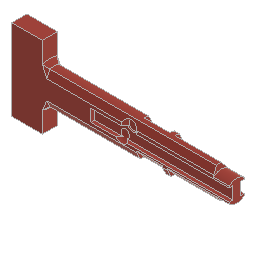
protec (Autodesk Fusion 360 design; units mm, degrees)
Autodesk Fusion 360 part; units mm, degrees
note: some values were not read from the file. Chosen so that the rebuilt part matches the saved one: which face or edge a step refers to; which pieces of a blend or face edit are solid.
sketch "profile" plane through (0, 0, 0) normal (1, 0, 0) x (0, 1, 0)
  line L0 (0, 0) -> (3.3, 0) construction
  line L1 (3.3, 0) -> (3.3, 3.3) construction
  line L2 (3.3, 3.3) -> (4.05, 3.3) construction
  line L3 (3.3, 3.3) -> (2.55, 3.3) construction
  line L4 (4.05, 3.3) -> (4.05, 4.5)
  line L5 (2.55, 3.3) -> (2.55, 2.1)
  line L6 (4.05, 3.3) -> (4.05, 2.1)
  line L7 (2.55, 3.3) -> (2.55, 4.5)
  line L8 (4.05, 4.5) -> (4.775, 4.5)
  line L9 (2.55, 2.1) -> (1.825, 2.1)
  line L10 (4.05, 2.1) -> (4.775, 2.1)
  line L11 (2.55, 4.5) -> (1.825, 4.5)
  line L12 (4.775, 4.5) -> (4.775, 5.165)
  line L13 (1.825, 2.1) -> (1.825, 1.435)
  line L14 (1.825, 4.5) -> (1.825, 5.165)
  line L15 (4.775, 2.1) -> (4.775, 1.435)
  line L16 (4.775, 5.165) -> (4.1589, 6.4863)
  line L17 (4.775, 5.165) -> (3.3, 5.165) construction
  line L18 (1.825, 1.435) -> (2.4411, 0.1137)
  line L19 (1.825, 5.165) -> (2.4411, 6.4863)
  line L20 (1.825, 5.165) -> (3.3, 5.165) construction
  line L21 (4.775, 1.435) -> (4.1589, 0.1137)
  arc A0 (4.1589, 6.4863) -> (2.4411, 6.4863) centre (3.3, 3.3) ccw
  arc A1 (2.4411, 0.1137) -> (4.1589, 0.1137) centre (3.3, 3.3) ccw
  dimension "d64" = 3.3
  dimension "d65" = 3.3
  dimension "d66" = 0.75
  dimension "d67" = 0.75
  dimension "d68" = 1.2
  dimension "d69" = 1.2
  dimension "d70" = 1.2
  dimension "d71" = 1.2
  dimension "d72" = 0.725
  dimension "d73" = 0.725
  dimension "d74" = 0.725
  dimension "d75" = 0.725
  dimension "d76" = 65
  dimension "d77" = 65
  dimension "d78" = 4.25
  dimension "d79" = 4.25
  dimension "d80" = 3.3
  constraint coincident L0.start origin
  constraint horizontal L0
  constraint perpendicular L0 L1
  constraint perpendicular L1 L2
  constraint perpendicular L1 L3
  constraint perpendicular L2 L4
  constraint perpendicular L3 L5
  constraint perpendicular L2 L6
  constraint perpendicular L3 L7
  constraint perpendicular L4 L8
  constraint perpendicular L5 L9
  constraint perpendicular L6 L10
  constraint perpendicular L7 L11
  constraint perpendicular L8 L12
  constraint perpendicular L9 L13
  constraint equal L12 L13
  constraint perpendicular L11 L14
  constraint perpendicular L10 L15
  constraint equal L14 L15
  constraint horizontal L17
  constraint vertical L1.end L17.end
  constraint equal L16 L18
  constraint parallel L16 L18
  constraint horizontal L20
  constraint parallel L19 L21
  constraint equal L19 L21
  constraint coincident L1.end L2.start
  constraint coincident L16.end A0.start
  measures "d64" distance of L0.start L0.end
  measures "d65" distance of L0.end L1.end
  measures "d66" distance of L1.end L2.end
  measures "d67" distance of L1.end L3.end
  measures "d68" distance of L2.end L4.end
  measures "d69" distance of L3.end L5.end
  measures "d70" distance of L2.end L6.end
  measures "d71" distance of L3.end L7.end
  measures "d72" distance of L4.end L8.end
  measures "d73" distance of L5.end L9.end
  measures "d74" distance of L6.end L10.end
  measures "d75" distance of L7.end L11.end
  measures "d76" angle of L16 L17
  measures "d77" angle of L19 L20
  measures "d78" distance of L16 L18
  measures "d79" distance of L19 L21
  measures "d80" radius of A0
extrude "Extrude1" add sketch "profile" against normal blind 42.57 makes body 1
ref_plane "WorkPlane1" through (-21.285, 3.3, 3.3) normal (0, -1, 0) x (0, 0, 1)
ref_plane "WorkPlane2" through (-42.57, 0, 0) normal (1, 0, 0) x (0, 1, 0)
sketch "bow" plane through (-42.57, 0, 0) normal (1, 0, 0) x (0, 1, 0)
  line L0 (2.55, 2.1) -> (2.55, 4.5)
  line L1 (2.55, 4.5) -> (1.825, 4.5)
  line L2 (1.825, 4.5) -> (1.825, 5.165) construction
  line L3 (1.825, 5.165) -> (2.4411, 6.4863) construction
  arc A0 (4.1589, 6.4863) -> (2.4411, 6.4863) centre (3.3, 3.3) ccw construction
  line L4 (4.1589, 6.4863) -> (4.775, 5.165) construction
  line L5 (4.775, 5.165) -> (4.775, 4.5) construction
  line L6 (4.775, 4.5) -> (4.05, 4.5)
  line L7 (4.05, 4.5) -> (4.05, 2.1)
  line L8 (4.05, 2.1) -> (4.775, 2.1)
  line L9 (4.775, 2.1) -> (4.775, 1.435) construction
  line L10 (4.775, 1.435) -> (4.1589, 0.1137) construction
  arc A1 (2.4411, 0.1137) -> (4.1589, 0.1137) centre (3.3, 3.3) ccw construction
  line L11 (2.4411, 0.1137) -> (1.825, 1.435) construction
  line L12 (1.825, 1.435) -> (1.825, 2.1) construction
  line L13 (1.825, 2.1) -> (2.55, 2.1)
  circle A2 centre (3.3, 3.3) radius 3.3 construction
  line L14 (1.825, 5.165) -> (1.825, 6.252)
  line L15 (1.825, 1.435) -> (1.825, 0.348)
  line L16 (4.775, 1.435) -> (4.775, 0.348)
  line L17 (4.775, 5.165) -> (4.775, 6.252)
  line L18 (1.825, 2.1) -> (1.825, 4.5)
  line L19 (4.775, 4.5) -> (4.775, 2.1)
  line L20 (1.825, 6.252) -> (1.825, 11.252)
  line L21 (4.775, 0.348) -> (4.775, -4.652)
  line L22 (1.825, 11.252) -> (4.775, 11.252)
  line L23 (4.775, 11.252) -> (4.775, 6.252)
  line L24 (4.775, -4.652) -> (1.825, -4.652)
  line L25 (1.825, -4.652) -> (1.825, 0.348)
  line L26 (1.825, 1.435) -> (1.825, 2.1)
  line L27 (4.775, 2.1) -> (4.775, 1.435)
  line L28 (4.775, 5.165) -> (4.775, 4.5)
  line L29 (1.825, 5.165) -> (1.825, 4.5)
  dimension "d84" = 5
  constraint concentric A0 A2
  constraint coincident L3.end A2
  constraint coincident L2.end L3.start
  constraint coincident A2 L14.end
  constraint parallel L2 L14
  constraint coincident L11.end L12.start
  constraint coincident A2 L15.end
  constraint parallel L12 L15
  constraint coincident L9.end L10.start
  constraint coincident A2 L16.end
  constraint parallel L9 L16
  constraint coincident L4.end L5.start
  constraint coincident A2 L17.end
  constraint parallel L5 L17
  constraint coincident L12.end L13.start
  constraint coincident L1.end L2.start
  constraint coincident L5.end L6.start
  constraint coincident L8.end L9.start
  constraint parallel L14 L20
  constraint parallel L16 L21
  constraint equal L20 L21
  constraint perpendicular L17 L22
  constraint perpendicular L22 L23
  constraint perpendicular L15 L24
  constraint perpendicular L24 L25
  measures "d84" distance of L14.end L20.end
sketch "dss holes + dc align" plane through (0, 3.3, 0) normal (0, -1, 0) x (-1, 0, 0)
  line L0 (0, -4.5) -> (0, -2.1) construction
  line L1 (0, -3.3) -> (19.57, -3.3) construction
  line L2 (19.57, -3.3) -> (21.07, -3.3) construction
  line L3 (19.57, -3.3) -> (19.57, -4.9) construction
  line L4 (19.57, -3.3) -> (19.57, -1.7) construction
  line L5 (21.07, -3.3) -> (21.07, -4.1) construction
  line L6 (21.07, -3.3) -> (21.07, -2.5) construction
  circle A0 centre (19.57, -4.9) radius 0.9
  circle A1 centre (16.57, -4.9) radius 0.9
  circle A2 centre (19.57, -1.7) radius 0.9
  circle A3 centre (16.57, -1.7) radius 0.9
  dimension "d85" = 19.57
  dimension "d86" = 1.5
  dimension "d87" = 1.6
  dimension "d88" = 0.8
  dimension "d89" = 1.8
  dimension "d90" = 3
  constraint midpoint L0 L1.start
  constraint perpendicular L0 L1
  constraint parallel L1 L2
  constraint perpendicular L2 L3
  constraint perpendicular L2 L4
  constraint equal L3 L4
  constraint perpendicular L2 L5
  constraint perpendicular L2 L6
  constraint equal L5 L6
  constraint coincident L3.end A0.centre
  constraint equal A0 A1
  constraint horizontal L3.end A1.centre
  constraint symmetric L1 A0 A2
  constraint symmetric L1 A1 A3
  measures "d85" distance of L1.start L1.end
  measures "d86" distance of L1.end L2.end
  measures "d87" distance of L1.end L3.end
  measures "d88" distance of L2.end L5.end
  measures "d89" diameter of A0
  measures "d90" distance of L3.end A1.centre
ref_plane "WorkPlane3" through (-21.07, 0, 0) normal (1, 0, 0) x (0, 1, 0)
sketch "dc bearings" plane through (-21.07, 0, 0) normal (1, 0, 0) x (0, 1, 0)
  line L0 (0, 0) -> (3.3, 0) construction
  line L1 (3.3, 0) -> (3.3, 3.3) construction
  line L2 (3.3, 3.3) -> (1.4542, 2.8398) construction
  line L3 (3.3, 3.3) -> (1.4542, 3.3) construction
  circle A0 centre (1.4542, 2.8398) radius 1.375
  line L4 (3.3, 3.3) -> (5.1458, 3.7602) construction
  circle A1 centre (5.1458, 3.7602) radius 1.375
  dimension "d92" = 3.3
  dimension "d93" = 3.3
  dimension "d94" = 14
  dimension "d95" = 1.9023
  dimension "d96" = 2.75
  constraint coincident L0.start origin
  constraint horizontal L0
  constraint perpendicular L0 L1
  constraint horizontal L3
  constraint coincident L2.end A0.centre
  constraint vertical L3.end L2.end
  constraint parallel L2 L4
  constraint equal L2 L4
  constraint coincident L4.end A1.centre
  constraint equal A0 A1
  measures "d92" distance of L0.start L0.end
  measures "d93" distance of L0.end L1.end
  measures "d94" angle of L2 L3
  measures "d95" distance of L1.end L2.end
  measures "d96" diameter of A0
extrude "Extrude2" add sketch "bow" along normal blind 6 bodies 1
extrude "Extrude3" add 2 faces at (-36.57, 2.0667, 3.7) (-36.57, 4.5333, 2.9) along direction (1, 0, 0) blind 9.5 on bodies 1 bodies 1
chamfer "Chamfer1" distance 0.85 angle 45 6 edges at (-36.57, 4.4669, 5.8256) (-36.57, 3.3, 6.6) (-36.57, 2.1331, 5.8256) (-36.57, 2.1331, 0.7744) (-36.57, 3.3, 0) (-36.57, 4.4669, 0.7744) on bodies 1
extrude "Extrude4" add sketch "dc bearings" along normal mid plane 2.75 separate body makes body 2 at (-20.1533, 6.5191, 3.6917) makes body 3 at (-20.1533, 2.8275, 2.7712)
fillet "Fillet1" radius 1.375 4 edges at (-19.695, 3.7708, 3.7602) (-22.445, 3.7708, 3.7602) (-19.695, 0.0792, 2.8398) (-22.445, 0.0792, 2.8398) on bodies 2 3
combine "Combine1" operation cut target body 1 tool bodies 2 3
extrude "Extrude5" cut sketch "dss holes + dc align" along normal blind 0.9 draft 35 from surface at 0.575 contours A0 bodies 1
extrude "Extrude6" cut sketch "dss holes + dc align" against normal blind 0.9 draft 35 from surface at -0.575 contours A2 bodies 1
extrude "Extrude17" [suppressed]
extrude "Extrude18" [suppressed]
sketch "profiled 0 cut" plane through (0, 0, 0) normal (1, 0, 0) x (0, 1, 0)
  line L0 (2.55, 4.5) -> (1.825, 4.5)
  line L1 (2.55, 3.3) -> (2.55, 4.5)
  line L2 (2.55, 3.3) -> (2.55, 2.1)
  line L3 (2.55, 2.1) -> (1.825, 2.1)
  line L4 (4.05, 3.3) -> (4.05, 2.1)
  line L5 (4.05, 2.1) -> (4.775, 2.1)
  line L6 (4.05, 3.3) -> (4.05, 4.5)
  line L7 (4.05, 4.5) -> (4.775, 4.5)
  line L8 (4.775, 4.5) -> (4.775, 4.8293)
  line L9 (1.825, 2.1) -> (1.825, 1.7707)
  line L10 (1.825, 4.5) -> (1.825, 4.8293)
  line L11 (4.775, 2.1) -> (4.775, 1.7707)
  line L12 (4.775, 4.8293) -> (4.7747, 4.83)
  line L13 (4.775, 4.8293) -> (3.3, 4.8293) construction
  line L14 (1.825, 1.7707) -> (1.8253, 1.77)
  line L15 (1.825, 4.8293) -> (1.8253, 4.83)
  line L16 (1.825, 4.8293) -> (3.3, 4.8293) construction
  line L17 (4.775, 1.7707) -> (4.7747, 1.77)
  arc A0 (4.7747, 4.83) -> (1.8253, 4.83) centre (3.3, 3.3) ccw
  arc A1 (1.8253, 1.77) -> (4.7747, 1.77) centre (3.3, 3.3) ccw
  circle A2 centre (3.3, 3.3) radius 4.125
  point P0 (3.3, 3.3)
  dimension "d112" = 65
  dimension "d113" = 65
  dimension "d114" = 2.125
  dimension "d115" = 3.9663
  dimension "d116" = 3.9663
  dimension "d117" = 8.25
  constraint coincident L7.end L8.start
  constraint perpendicular L7 L8
  constraint coincident L3.end L9.start
  constraint perpendicular L3 L9
  constraint equal L8 L9
  constraint coincident L0.end L10.start
  constraint perpendicular L0 L10
  constraint coincident L5.end L11.start
  constraint perpendicular L5 L11
  constraint equal L10 L11
  constraint horizontal L13
  constraint vertical P0 L13.end
  constraint parallel L12 L14
  constraint equal L12 L14
  constraint horizontal L16
  constraint parallel L15 L17
  constraint equal L15 L17
  constraint coincident P0 A0.centre
  constraint coincident L12.end A0.start
  constraint equal A0 A1
  constraint concentric A0 A2
  measures "d112" angle of L12 L13
  measures "d113" angle of L15 L16
  measures "d114" radius of A0
  measures "d115" distance of L15 L17
  measures "d116" distance of L12 L14
  measures "d117" diameter of A2
sketch "Sketch6" plane through (0, 0, 0) normal (1, 0, 0) x (0, 1, 0)
  line L0 (2.55, 2.1) -> (1.825, 2.1)
  line L1 (2.55, 3.3) -> (2.55, 2.1)
  line L2 (2.55, 3.3) -> (2.55, 4.5)
  line L3 (2.55, 4.5) -> (1.825, 4.5)
  line L4 (4.05, 4.5) -> (4.775, 4.5)
  line L5 (4.05, 3.3) -> (4.05, 4.5)
  line L6 (4.05, 3.3) -> (4.05, 2.1)
  line L7 (4.05, 2.1) -> (4.775, 2.1)
  line L8 (4.775, 4.5) -> (4.775, 4.8481)
  line L9 (1.825, 2.1) -> (1.825, 1.7519)
  line L10 (1.825, 4.5) -> (1.825, 5.165)
  line L11 (4.775, 2.1) -> (4.775, 1.435)
  line L12 (4.775, 4.8481) -> (3.305, 6.6)
  line L13 (4.775, 4.8481) -> (3.3, 4.8481) construction
  line L14 (1.825, 1.7519) -> (3.295, 0)
  line L15 (1.825, 5.165) -> (2.4411, 6.4863)
  line L16 (1.825, 5.165) -> (3.3, 5.165) construction
  line L17 (4.775, 1.435) -> (4.1589, 0.1137)
  arc A0 (3.305, 6.6) -> (2.4411, 6.4863) centre (3.3, 3.3) ccw
  arc A1 (3.295, 0) -> (4.1589, 0.1137) centre (3.3, 3.3) ccw
  circle A2 centre (3.3, 3.3) radius 4.125
  point P0 (3.3, 3.3)
  dimension "d118" = 50
  dimension "d119" = 65
  dimension "d120" = 3.3
  dimension "d121" = 4.25
  dimension "d122" = 4.25
  dimension "d123" = 8.25
  constraint coincident L4.end L8.start
  constraint perpendicular L4 L8
  constraint coincident L0.end L9.start
  constraint perpendicular L0 L9
  constraint equal L8 L9
  constraint coincident L3.end L10.start
  constraint perpendicular L3 L10
  constraint coincident L7.end L11.start
  constraint perpendicular L7 L11
  constraint equal L10 L11
  constraint horizontal L13
  constraint vertical P0 L13.end
  constraint parallel L12 L14
  constraint equal L12 L14
  constraint horizontal L16
  constraint vertical P0 L16.end
  constraint parallel L15 L17
  constraint equal L15 L17
  constraint coincident P0 A0.centre
  constraint coincident L12.end A0.start
  constraint equal A0 A1
  constraint concentric A1 A2
  measures "d118" angle of L12 L13
  measures "d119" angle of L15 L16
  measures "d120" radius of A0
  measures "d121" distance of L12 L14
  measures "d122" distance of L15 L17
  measures "d123" diameter of A2
sketch "Sketch7" plane through (0, 0, 0) normal (1, 0, 0) x (0, 1, 0)
  line L0 (4.05, 4.5) -> (4.775, 4.5)
  line L1 (4.05, 3.3) -> (4.05, 4.5)
  line L2 (4.05, 3.3) -> (4.05, 2.1)
  line L3 (4.05, 2.1) -> (4.775, 2.1)
  line L4 (2.55, 2.1) -> (1.825, 2.1)
  line L5 (2.55, 3.3) -> (2.55, 2.1)
  line L6 (2.55, 3.3) -> (2.55, 4.5)
  line L7 (2.55, 4.5) -> (1.825, 4.5)
  line L8 (4.775, 4.5) -> (4.775, 4.8481)
  line L9 (1.825, 2.1) -> (1.825, 1.7519)
  line L10 (1.825, 4.5) -> (1.825, 5.165)
  line L11 (4.775, 2.1) -> (4.775, 1.435)
  line L12 (4.775, 4.8481) -> (3.305, 6.6)
  line L13 (4.775, 4.8481) -> (3.3, 4.8481) construction
  line L14 (1.825, 1.7519) -> (3.295, 0)
  line L15 (1.825, 5.165) -> (2.4411, 6.4863)
  line L16 (1.825, 5.165) -> (3.3, 5.165) construction
  line L17 (4.775, 1.435) -> (4.1589, 0.1137)
  arc A0 (3.305, 6.6) -> (2.4411, 6.4863) centre (3.3, 3.3) ccw
  arc A1 (3.295, 0) -> (4.1589, 0.1137) centre (3.3, 3.3) ccw
  circle A2 centre (3.3, 3.3) radius 4.125
  point P0 (3.3, 3.3)
  dimension "d124" = 50
  dimension "d125" = 65
  dimension "d126" = 3.3
  dimension "d127" = 4.25
  dimension "d128" = 4.25
  dimension "d129" = 8.25
  constraint coincident L0.end L8.start
  constraint perpendicular L0 L8
  constraint coincident L4.end L9.start
  constraint perpendicular L4 L9
  constraint coincident L7.end L10.start
  constraint perpendicular L7 L10
  constraint coincident L3.end L11.start
  constraint perpendicular L3 L11
  constraint equal L8 L9
  constraint equal L10 L11
  constraint horizontal L13
  constraint vertical P0 L13.end
  constraint parallel L12 L14
  constraint equal L12 L14
  constraint horizontal L16
  constraint vertical P0 L16.end
  constraint parallel L15 L17
  constraint equal L15 L17
  constraint coincident P0 A0.centre
  constraint coincident L12.end A0.start
  constraint equal A0 A1
  constraint concentric A1 A2
  measures "d124" angle of L12 L13
  measures "d125" angle of L15 L16
  measures "d126" radius of A0
  measures "d127" distance of L12 L14
  measures "d128" distance of L15 L17
  measures "d129" diameter of A2
sketch "Sketch8" plane through (0, 0, 0) normal (1, 0, 0) x (0, 1, 0)
  line L0 (2.55, 4.5) -> (1.825, 4.5)
  line L1 (2.55, 3.3) -> (2.55, 4.5)
  line L2 (2.55, 3.3) -> (2.55, 2.1)
  line L3 (2.55, 2.1) -> (1.825, 2.1)
  line L4 (4.05, 4.5) -> (4.775, 4.5)
  line L5 (4.05, 3.3) -> (4.05, 4.5)
  line L6 (4.05, 3.3) -> (4.05, 2.1)
  line L7 (4.05, 2.1) -> (4.775, 2.1)
  line L8 (4.775, 4.5) -> (4.775, 4.8481)
  line L9 (1.825, 2.1) -> (1.825, 1.7519)
  line L10 (1.825, 4.5) -> (1.825, 5.165)
  line L11 (4.775, 2.1) -> (4.775, 1.435)
  line L12 (4.775, 4.8481) -> (3.305, 6.6)
  line L13 (4.775, 4.8481) -> (3.3, 4.8481) construction
  line L14 (1.825, 1.7519) -> (3.295, 0)
  line L15 (1.825, 5.165) -> (2.4411, 6.4863)
  line L16 (1.825, 5.165) -> (3.3, 5.165) construction
  line L17 (4.775, 1.435) -> (4.1589, 0.1137)
  arc A0 (3.305, 6.6) -> (2.4411, 6.4863) centre (3.3, 3.3) ccw
  arc A1 (3.295, 0) -> (4.1589, 0.1137) centre (3.3, 3.3) ccw
  circle A2 centre (3.3, 3.3) radius 4.125
  point P0 (3.3, 3.3)
  dimension "d130" = 50
  dimension "d131" = 65
  dimension "d132" = 3.3
  dimension "d133" = 4.25
  dimension "d134" = 4.25
  dimension "d135" = 8.25
  constraint coincident L4.end L8.start
  constraint perpendicular L4 L8
  constraint coincident L3.end L9.start
  constraint perpendicular L3 L9
  constraint coincident L0.end L10.start
  constraint perpendicular L0 L10
  constraint coincident L7.end L11.start
  constraint perpendicular L7 L11
  constraint equal L8 L9
  constraint equal L10 L11
  constraint horizontal L13
  constraint vertical P0 L13.end
  constraint parallel L12 L14
  constraint equal L12 L14
  constraint horizontal L16
  constraint vertical P0 L16.end
  constraint parallel L15 L17
  constraint equal L15 L17
  constraint coincident P0 A0.centre
  constraint coincident L12.end A0.start
  constraint equal A0 A1
  constraint concentric A0 A2
  measures "d130" angle of L12 L13
  measures "d131" angle of L15 L16
  measures "d132" radius of A0
  measures "d133" distance of L12 L14
  measures "d134" distance of L15 L17
  measures "d135" diameter of A2
sketch "Sketch9" plane through (0, 0, 0) normal (1, 0, 0) x (0, 1, 0)
  line L0 (2.55, 4.5) -> (1.825, 4.5)
  line L1 (2.55, 3.3) -> (2.55, 4.5)
  line L2 (2.55, 3.3) -> (2.55, 2.1)
  line L3 (2.55, 2.1) -> (1.825, 2.1)
  line L4 (4.05, 4.5) -> (4.775, 4.5)
  line L5 (4.05, 3.3) -> (4.05, 4.5)
  line L6 (4.05, 3.3) -> (4.05, 2.1)
  line L7 (4.05, 2.1) -> (4.775, 2.1)
  line L8 (4.775, 4.5) -> (4.775, 4.8481)
  line L9 (1.825, 2.1) -> (1.825, 1.7519)
  line L10 (1.825, 4.5) -> (1.825, 5.165)
  line L11 (4.775, 2.1) -> (4.775, 1.435)
  line L12 (4.775, 4.8481) -> (3.305, 6.6)
  line L13 (4.775, 4.8481) -> (3.3, 4.8481) construction
  line L14 (1.825, 1.7519) -> (3.295, 0)
  line L15 (1.825, 5.165) -> (2.4411, 6.4863)
  line L16 (1.825, 5.165) -> (3.3, 5.165) construction
  line L17 (4.775, 1.435) -> (4.1589, 0.1137)
  arc A0 (3.305, 6.6) -> (2.4411, 6.4863) centre (3.3, 3.3) ccw
  arc A1 (3.295, 0) -> (4.1589, 0.1137) centre (3.3, 3.3) ccw
  circle A2 centre (3.3, 3.3) radius 4.125
  point P0 (3.3, 3.3)
  dimension "d136" = 50
  dimension "d137" = 65
  dimension "d138" = 3.3
  dimension "d139" = 4.25
  dimension "d140" = 4.25
  dimension "d141" = 8.25
  constraint coincident L4.end L8.start
  constraint perpendicular L4 L8
  constraint coincident L3.end L9.start
  constraint perpendicular L3 L9
  constraint coincident L0.end L10.start
  constraint perpendicular L0 L10
  constraint coincident L7.end L11.start
  constraint perpendicular L7 L11
  constraint equal L8 L9
  constraint equal L10 L11
  constraint horizontal L13
  constraint vertical P0 L13.end
  constraint parallel L12 L14
  constraint equal L12 L14
  constraint horizontal L16
  constraint vertical P0 L16.end
  constraint parallel L15 L17
  constraint equal L15 L17
  constraint coincident P0 A0.centre
  constraint coincident L12.end A0.start
  constraint equal A0 A1
  measures "d136" angle of L12 L13
  measures "d137" angle of L15 L16
  measures "d138" radius of A0
  measures "d139" distance of L12 L14
  measures "d140" distance of L15 L17
  measures "d141" diameter of A2
sketch "Sketch10" plane through (0, 0, 0) normal (1, 0, 0) x (0, 1, 0)
  line L0 (2.55, 4.5) -> (1.825, 4.5)
  line L1 (2.55, 3.3) -> (2.55, 4.5)
  line L2 (2.55, 3.3) -> (2.55, 2.1)
  line L3 (2.55, 2.1) -> (1.825, 2.1)
  line L4 (4.05, 4.5) -> (4.775, 4.5)
  line L5 (4.05, 3.3) -> (4.05, 4.5)
  line L6 (4.05, 3.3) -> (4.05, 2.1)
  line L7 (4.05, 2.1) -> (4.775, 2.1)
  line L8 (4.775, 4.5) -> (4.775, 4.8481)
  line L9 (1.825, 2.1) -> (1.825, 1.7519)
  line L10 (1.825, 4.5) -> (1.825, 5.165)
  line L11 (4.775, 2.1) -> (4.775, 1.435)
  line L12 (4.775, 4.8481) -> (3.305, 6.6)
  line L13 (4.775, 4.8481) -> (3.3, 4.8481) construction
  line L14 (1.825, 1.7519) -> (3.295, 0)
  line L15 (1.825, 5.165) -> (2.4411, 6.4863)
  line L16 (1.825, 5.165) -> (3.3, 5.165) construction
  line L17 (4.775, 1.435) -> (4.1589, 0.1137)
  arc A0 (3.305, 6.6) -> (2.4411, 6.4863) centre (3.3, 3.3) ccw
  arc A1 (3.295, 0) -> (4.1589, 0.1137) centre (3.3, 3.3) ccw
  circle A2 centre (3.3, 3.3) radius 4.125
  point P0 (3.3, 3.3)
  dimension "d142" = 50
  dimension "d143" = 65
  dimension "d144" = 3.3
  dimension "d145" = 4.25
  dimension "d146" = 4.25
  dimension "d147" = 8.25
  constraint coincident L4.end L8.start
  constraint perpendicular L4 L8
  constraint coincident L3.end L9.start
  constraint perpendicular L3 L9
  constraint coincident L0.end L10.start
  constraint perpendicular L0 L10
  constraint coincident L7.end L11.start
  constraint perpendicular L7 L11
  constraint equal L8 L9
  constraint equal L10 L11
  constraint horizontal L13
  constraint vertical P0 L13.end
  constraint parallel L12 L14
  constraint equal L12 L14
  constraint horizontal L16
  constraint vertical P0 L16.end
  constraint parallel L15 L17
  constraint equal L15 L17
  constraint coincident P0 A0.centre
  constraint coincident L12.end A0.start
  constraint equal A0 A1
  constraint concentric A0 A2
  measures "d142" angle of L12 L13
  measures "d143" angle of L15 L16
  measures "d144" radius of A0
  measures "d145" distance of L12 L14
  measures "d146" distance of L15 L17
  measures "d147" diameter of A2
sketch "Sketch11" plane through (0, 0, 0) normal (1, 0, 0) x (0, 1, 0)
  line L0 (2.55, 4.5) -> (1.825, 4.5)
  line L1 (2.55, 3.3) -> (2.55, 4.5)
  line L2 (2.55, 3.3) -> (2.55, 2.1)
  line L3 (2.55, 2.1) -> (1.825, 2.1)
  line L4 (4.05, 4.5) -> (4.775, 4.5)
  line L5 (4.05, 3.3) -> (4.05, 4.5)
  line L6 (4.05, 3.3) -> (4.05, 2.1)
  line L7 (4.05, 2.1) -> (4.775, 2.1)
  line L8 (4.775, 4.5) -> (4.775, 4.8481)
  line L9 (1.825, 2.1) -> (1.825, 1.7519)
  line L10 (1.825, 4.5) -> (1.825, 5.165)
  line L11 (4.775, 2.1) -> (4.775, 1.435)
  line L12 (4.775, 4.8481) -> (3.305, 6.6)
  line L13 (4.775, 4.8481) -> (3.3, 4.8481) construction
  line L14 (1.825, 1.7519) -> (3.295, 0)
  line L15 (1.825, 5.165) -> (2.4411, 6.4863)
  line L16 (1.825, 5.165) -> (3.3, 5.165) construction
  line L17 (4.775, 1.435) -> (4.1589, 0.1137)
  arc A0 (3.305, 6.6) -> (2.4411, 6.4863) centre (3.3, 3.3) ccw
  arc A1 (3.295, 0) -> (4.1589, 0.1137) centre (3.3, 3.3) ccw
  circle A2 centre (3.3, 3.3) radius 4.125
  point P0 (3.3, 3.3)
  dimension "d148" = 50
  dimension "d149" = 65
  dimension "d150" = 3.3
  dimension "d151" = 4.25
  dimension "d152" = 4.25
  dimension "d153" = 8.25
  constraint coincident L4.end L8.start
  constraint perpendicular L4 L8
  constraint coincident L3.end L9.start
  constraint perpendicular L3 L9
  constraint coincident L0.end L10.start
  constraint perpendicular L0 L10
  constraint coincident L7.end L11.start
  constraint perpendicular L7 L11
  constraint equal L8 L9
  constraint equal L10 L11
  constraint horizontal L13
  constraint vertical P0 L13.end
  constraint parallel L12 L14
  constraint equal L12 L14
  constraint horizontal L16
  constraint vertical P0 L16.end
  constraint parallel L15 L17
  constraint equal L15 L17
  constraint coincident P0 A0.centre
  constraint coincident L12.end A0.start
  constraint equal A0 A1
  constraint concentric A1 A2
  measures "d148" angle of L12 L13
  measures "d149" angle of L15 L16
  measures "d150" radius of A0
  measures "d151" distance of L12 L14
  measures "d152" distance of L15 L17
  measures "d153" diameter of A2
sketch "Sketch12" plane through (0, 0, 0) normal (1, 0, 0) x (0, 1, 0)
  line L0 (2.55, 4.5) -> (1.825, 4.5)
  line L1 (2.55, 3.3) -> (2.55, 4.5)
  line L2 (2.55, 3.3) -> (2.55, 2.1)
  line L3 (2.55, 2.1) -> (1.825, 2.1)
  line L4 (4.05, 4.5) -> (4.775, 4.5)
  line L5 (4.05, 3.3) -> (4.05, 4.5)
  line L6 (4.05, 3.3) -> (4.05, 2.1)
  line L7 (4.05, 2.1) -> (4.775, 2.1)
  line L8 (4.775, 4.5) -> (4.775, 4.8481)
  line L9 (1.825, 2.1) -> (1.825, 1.7519)
  line L10 (1.825, 4.5) -> (1.825, 5.165)
  line L11 (4.775, 2.1) -> (4.775, 1.435)
  line L12 (4.775, 4.8481) -> (3.305, 6.6)
  line L13 (4.775, 4.8481) -> (3.3, 4.8481) construction
  line L14 (1.825, 1.7519) -> (3.295, 0)
  line L15 (1.825, 5.165) -> (2.4411, 6.4863)
  line L16 (1.825, 5.165) -> (3.3, 5.165) construction
  line L17 (4.775, 1.435) -> (4.1589, 0.1137)
  arc A0 (3.305, 6.6) -> (2.4411, 6.4863) centre (3.3, 3.3) ccw
  arc A1 (3.295, 0) -> (4.1589, 0.1137) centre (3.3, 3.3) ccw
  circle A2 centre (3.3, 3.3) radius 4.125
  point P0 (3.3, 3.3)
  dimension "d154" = 50
  dimension "d155" = 65
  dimension "d156" = 3.3
  dimension "d157" = 4.25
  dimension "d158" = 4.25
  dimension "d159" = 8.25
  constraint coincident L4.end L8.start
  constraint perpendicular L4 L8
  constraint coincident L3.end L9.start
  constraint perpendicular L3 L9
  constraint coincident L0.end L10.start
  constraint perpendicular L0 L10
  constraint coincident L7.end L11.start
  constraint perpendicular L7 L11
  constraint equal L8 L9
  constraint equal L10 L11
  constraint horizontal L13
  constraint vertical P0 L13.end
  constraint parallel L12 L14
  constraint equal L12 L14
  constraint horizontal L16
  constraint vertical P0 L16.end
  constraint parallel L15 L17
  constraint equal L15 L17
  constraint coincident P0 A0.centre
  constraint coincident L12.end A0.start
  constraint equal A0 A1
  constraint concentric A0 A2
  measures "d154" angle of L12 L13
  measures "d155" angle of L15 L16
  measures "d156" radius of A0
  measures "d157" distance of L12 L14
  measures "d158" distance of L15 L17
  measures "d159" diameter of A2
sketch "Sketch13" plane through (0, 0, 0) normal (1, 0, 0) x (0, 1, 0)
  line L0 (2.55, 4.5) -> (1.825, 4.5)
  line L1 (2.55, 3.3) -> (2.55, 4.5)
  line L2 (2.55, 3.3) -> (2.55, 2.1)
  line L3 (2.55, 2.1) -> (1.825, 2.1)
  line L4 (4.05, 4.5) -> (4.775, 4.5)
  line L5 (4.05, 3.3) -> (4.05, 4.5)
  line L6 (4.05, 3.3) -> (4.05, 2.1)
  line L7 (4.05, 2.1) -> (4.775, 2.1)
  line L8 (4.775, 4.5) -> (4.775, 4.8481)
  line L9 (1.825, 2.1) -> (1.825, 1.7519)
  line L10 (1.825, 4.5) -> (1.825, 5.165)
  line L11 (4.775, 2.1) -> (4.775, 1.435)
  line L12 (4.775, 4.8481) -> (3.305, 6.6)
  line L13 (4.775, 4.8481) -> (3.3, 4.8481) construction
  line L14 (1.825, 1.7519) -> (3.295, 0)
  line L15 (1.825, 5.165) -> (2.4411, 6.4863)
  line L16 (1.825, 5.165) -> (3.3, 5.165) construction
  line L17 (4.775, 1.435) -> (4.1589, 0.1137)
  arc A0 (3.305, 6.6) -> (2.4411, 6.4863) centre (3.3, 3.3) ccw
  arc A1 (3.295, 0) -> (4.1589, 0.1137) centre (3.3, 3.3) ccw
  circle A2 centre (3.3, 3.3) radius 4.125
  point P0 (3.3, 3.3)
  dimension "d160" = 50
  dimension "d161" = 65
  dimension "d162" = 3.3
  dimension "d163" = 4.25
  dimension "d164" = 4.25
  dimension "d165" = 8.25
  constraint coincident L4.end L8.start
  constraint perpendicular L4 L8
  constraint coincident L3.end L9.start
  constraint perpendicular L3 L9
  constraint coincident L0.end L10.start
  constraint perpendicular L0 L10
  constraint coincident L7.end L11.start
  constraint perpendicular L7 L11
  constraint equal L8 L9
  constraint equal L10 L11
  constraint horizontal L13
  constraint vertical P0 L13.end
  constraint parallel L12 L14
  constraint equal L12 L14
  constraint horizontal L16
  constraint vertical P0 L16.end
  constraint parallel L15 L17
  constraint equal L15 L17
  constraint coincident P0 A0.centre
  constraint coincident L12.end A0.start
  constraint equal A0 A1
  constraint concentric A0 A2
  measures "d160" angle of L12 L13
  measures "d161" angle of L15 L16
  measures "d162" radius of A0
  measures "d163" distance of L12 L14
  measures "d164" distance of L15 L17
  measures "d165" diameter of A2
sketch "Sketch14" plane through (0, 0, 0) normal (1, 0, 0) x (0, 1, 0)
  line L0 (2.55, 4.5) -> (1.825, 4.5)
  line L1 (2.55, 3.3) -> (2.55, 4.5)
  line L2 (2.55, 3.3) -> (2.55, 2.1)
  line L3 (2.55, 2.1) -> (1.825, 2.1)
  line L4 (4.05, 4.5) -> (4.775, 4.5)
  line L5 (4.05, 3.3) -> (4.05, 4.5)
  line L6 (4.05, 3.3) -> (4.05, 2.1)
  line L7 (4.05, 2.1) -> (4.775, 2.1)
  line L8 (4.775, 4.5) -> (4.775, 4.8481)
  line L9 (1.825, 2.1) -> (1.825, 1.7519)
  line L10 (1.825, 4.5) -> (1.825, 5.165)
  line L11 (4.775, 2.1) -> (4.775, 1.435)
  line L12 (4.775, 4.8481) -> (3.305, 6.6)
  line L13 (4.775, 4.8481) -> (3.3, 4.8481) construction
  line L14 (1.825, 1.7519) -> (3.295, 0)
  line L15 (1.825, 5.165) -> (2.4411, 6.4863)
  line L16 (1.825, 5.165) -> (3.3, 5.165) construction
  line L17 (4.775, 1.435) -> (4.1589, 0.1137)
  arc A0 (3.305, 6.6) -> (2.4411, 6.4863) centre (3.3, 3.3) ccw
  arc A1 (3.295, 0) -> (4.1589, 0.1137) centre (3.3, 3.3) ccw
  circle A2 centre (3.3, 3.3) radius 4.125
  point P0 (3.3, 3.3)
  dimension "d166" = 50
  dimension "d167" = 65
  dimension "d168" = 3.3
  dimension "d169" = 4.25
  dimension "d170" = 4.25
  dimension "d171" = 8.25
  constraint coincident L4.end L8.start
  constraint perpendicular L4 L8
  constraint coincident L3.end L9.start
  constraint perpendicular L3 L9
  constraint coincident L0.end L10.start
  constraint perpendicular L0 L10
  constraint coincident L7.end L11.start
  constraint perpendicular L7 L11
  constraint equal L8 L9
  constraint equal L10 L11
  constraint horizontal L13
  constraint vertical P0 L13.end
  constraint parallel L12 L14
  constraint equal L12 L14
  constraint horizontal L16
  constraint vertical P0 L16.end
  constraint parallel L15 L17
  constraint equal L15 L17
  constraint coincident P0 A0.centre
  constraint coincident L12.end A0.start
  constraint equal A0 A1
  constraint concentric A1 A2
  measures "d166" angle of L12 L13
  measures "d167" angle of L15 L16
  measures "d168" radius of A0
  measures "d169" distance of L12 L14
  measures "d170" distance of L15 L17
  measures "d171" diameter of A2
extrude "Extrude7" cut sketch "profiled 0 cut" against normal blind 3.07 bodies 1
extrude "Extrude8" cut sketch "Sketch6" along normal mid plane 2 from surface at -3.57 bodies 1
extrude "Extrude9" cut sketch "Sketch7" along normal mid plane 2 from surface at -5.07 bodies 1
extrude "Extrude10" cut sketch "Sketch8" along normal mid plane 2 from surface at -6.57 bodies 1
extrude "Extrude11" cut sketch "Sketch9" along normal mid plane 2 from surface at -8.07 bodies 1
extrude "Extrude12" cut sketch "Sketch10" along normal mid plane 2 from surface at -9.57 bodies 1
extrude "Extrude13" cut sketch "Sketch11" along normal mid plane 2 from surface at -11.07 bodies 1
extrude "Extrude14" cut sketch "Sketch12" along normal mid plane 2 from surface at -14.07 bodies 1
extrude "Extrude15" cut sketch "Sketch13" along normal mid plane 2 from surface at -15.57 bodies 1
extrude "Extrude16" cut sketch "Sketch14" along normal mid plane 2 from surface at -17.07 bodies 1
equation "pos_1 = round($1)"
equation "cut_1 = if(pos_1 == 1; 1; if(pos_1 == 2; 2; if(pos_1 == 3; 3; if(pos_1 == 4; 4; if(pos_1 == 5; 5; 6)))))"
equation "right_angle_1 = if(cut_1 == 1; 50 deg; if(cut_1 == 2; 65 deg; if(cut_1 == 3; 35 deg; if(cut_1 == 4; 50 deg; if(cut_1 == 5; 65 deg; 65 deg)))))"
equation "left_angle_1 = if(cut_1 == 1; 65 deg; if(cut_1 == 2; 50 deg; if(cut_1 == 3; 65 deg; if(cut_1 == 4; 50 deg; if(cut_1 == 5; 35 deg; 65 deg)))))"
equation "end_diameters_1 = if(( cut_1 == 1 ) or ( cut_1 == 2 ); 3.3 mm; if(( cut_1 == 3 ) or ( cut_1 == 4 ) or ( cut_1 == 5 ); 2.7 mm; 2.125 mm))"
equation "parallel_distance_1 = if(( cut_1 == 1 ) or ( cut_1 == 2 ) or ( cut_1 == 3 ) or ( cut_1 == 4 ) or ( cut_1 == 5 ); 4.25 mm; 3.96625 mm)"
equation "pos_2 = round($2)"
equation "cut_2 = if(pos_2 == 1; 1; if(pos_2 == 2; 2; if(pos_2 == 3; 3; if(pos_2 == 4; 4; if(pos_2 == 5; 5; 6)))))"
equation "right_angle_2 = if(cut_2 == 1; 50 deg; if(cut_2 == 2; 65 deg; if(cut_2 == 3; 35 deg; if(cut_2 == 4; 50 deg; if(cut_2 == 5; 65 deg; 65 deg)))))"
equation "left_angle_2 = if(cut_2 == 1; 65 deg; if(cut_2 == 2; 50 deg; if(cut_2 == 3; 65 deg; if(cut_2 == 4; 50 deg; if(cut_2 == 5; 35 deg; 65 deg)))))"
equation "end_diameters_2 = if(( cut_2 == 1 ) or ( cut_2 == 2 ); 3.3 mm; if(( cut_2 == 3 ) or ( cut_2 == 4 ) or ( cut_2 == 5 ); 2.7 mm; 2.125 mm))"
equation "parallel_distance_2 = if(( cut_2 == 1 ) or ( cut_2 == 2 ) or ( cut_2 == 3 ) or ( cut_2 == 4 ) or ( cut_2 == 5 ); 4.25 mm; 3.96625 mm)"
equation "pos_3 = round($3)"
equation "cut_3 = if(pos_3 == 1; 1; if(pos_3 == 2; 2; if(pos_3 == 3; 3; if(pos_3 == 4; 4; if(pos_3 == 5; 5; 6)))))"
equation "right_angle_3 = if(cut_3 == 1; 50 deg; if(cut_3 == 2; 65 deg; if(cut_3 == 3; 35 deg; if(cut_3 == 4; 50 deg; if(cut_3 == 5; 65 deg; 65 deg)))))"
equation "left_angle_3 = if(cut_3 == 1; 65 deg; if(cut_3 == 2; 50 deg; if(cut_3 == 3; 65 deg; if(cut_3 == 4; 50 deg; if(cut_3 == 5; 35 deg; 65 deg)))))"
equation "end_diameters_3 = if(( cut_3 == 1 ) or ( cut_3 == 2 ); 3.3 mm; if(( cut_3 == 3 ) or ( cut_3 == 4 ) or ( cut_3 == 5 ); 2.7 mm; 2.125 mm))"
equation "parallel_distance_3 = if(( cut_3 == 1 ) or ( cut_3 == 2 ) or ( cut_3 == 3 ) or ( cut_3 == 4 ) or ( cut_3 == 5 ); 4.25 mm; 3.96625 mm)"
equation "pos_4 = round($4)"
equation "cut_4 = if(pos_4 == 1; 1; if(pos_4 == 2; 2; if(pos_4 == 3; 3; if(pos_4 == 4; 4; if(pos_4 == 5; 5; 6)))))"
equation "right_angle_4 = if(cut_4 == 1; 50 deg; if(cut_4 == 2; 65 deg; if(cut_4 == 3; 35 deg; if(cut_4 == 4; 50 deg; if(cut_4 == 5; 65 deg; 65 deg)))))"
equation "left_angle_4 = if(cut_4 == 1; 65 deg; if(cut_4 == 2; 50 deg; if(cut_4 == 3; 65 deg; if(cut_4 == 4; 50 deg; if(cut_4 == 5; 35 deg; 65 deg)))))"
equation "end_diameters_4 = if(( cut_4 == 1 ) or ( cut_4 == 2 ); 3.3 mm; if(( cut_4 == 3 ) or ( cut_4 == 4 ) or ( cut_4 == 5 ); 2.7 mm; 2.125 mm))"
equation "parallel_distance_4 = if(( cut_4 == 1 ) or ( cut_4 == 2 ) or ( cut_4 == 3 ) or ( cut_4 == 4 ) or ( cut_4 == 5 ); 4.25 mm; 3.96625 mm)"
equation "pos_5 = round($5)"
equation "cut_5 = if(pos_5 == 1; 1; if(pos_5 == 2; 2; if(pos_5 == 3; 3; if(pos_5 == 4; 4; if(pos_5 == 5; 5; 6)))))"
equation "right_angle_5 = if(cut_5 == 1; 50 deg; if(cut_5 == 2; 65 deg; if(cut_5 == 3; 35 deg; if(cut_5 == 4; 50 deg; if(cut_5 == 5; 65 deg; 65 deg)))))"
equation "left_angle_5 = if(cut_5 == 1; 65 deg; if(cut_5 == 2; 50 deg; if(cut_5 == 3; 65 deg; if(cut_5 == 4; 50 deg; if(cut_5 == 5; 35 deg; 65 deg)))))"
equation "end_diameters_5 = if(( cut_5 == 1 ) or ( cut_5 == 2 ); 3.3 mm; if(( cut_5 == 3 ) or ( cut_5 == 4 ) or ( cut_5 == 5 ); 2.7 mm; 2.125 mm))"
equation "parallel_distance_5 = if(( cut_5 == 1 ) or ( cut_5 == 2 ) or ( cut_5 == 3 ) or ( cut_5 == 4 ) or ( cut_5 == 5 ); 4.25 mm; 3.96625 mm)"
equation "pos_6 = round($6)"
equation "cut_6 = if(pos_6 == 1; 1; if(pos_6 == 2; 2; if(pos_6 == 3; 3; if(pos_6 == 4; 4; if(pos_6 == 5; 5; 6)))))"
equation "right_angle_6 = if(cut_6 == 1; 50 deg; if(cut_6 == 2; 65 deg; if(cut_6 == 3; 35 deg; if(cut_6 == 4; 50 deg; if(cut_6 == 5; 65 deg; 65 deg)))))"
equation "left_angle_6 = if(cut_6 == 1; 65 deg; if(cut_6 == 2; 50 deg; if(cut_6 == 3; 65 deg; if(cut_6 == 4; 50 deg; if(cut_6 == 5; 35 deg; 65 deg)))))"
equation "end_diameters_6 = if(( cut_6 == 1 ) or ( cut_6 == 2 ); 3.3 mm; if(( cut_6 == 3 ) or ( cut_6 == 4 ) or ( cut_6 == 5 ); 2.7 mm; 2.125 mm))"
equation "parallel_distance_6 = if(( cut_6 == 1 ) or ( cut_6 == 2 ) or ( cut_6 == 3 ) or ( cut_6 == 4 ) or ( cut_6 == 5 ); 4.25 mm; 3.96625 mm)"
equation "pos_7 = round($7)"
equation "cut_7 = if(pos_7 == 1; 1; if(pos_7 == 2; 2; if(pos_7 == 3; 3; if(pos_7 == 4; 4; if(pos_7 == 5; 5; 6)))))"
equation "right_angle_7 = if(cut_7 == 1; 50 deg; if(cut_7 == 2; 65 deg; if(cut_7 == 3; 35 deg; if(cut_7 == 4; 50 deg; if(cut_7 == 5; 65 deg; 65 deg)))))"
equation "left_angle_7 = if(cut_7 == 1; 65 deg; if(cut_7 == 2; 50 deg; if(cut_7 == 3; 65 deg; if(cut_7 == 4; 50 deg; if(cut_7 == 5; 35 deg; 65 deg)))))"
equation "end_diameters_7 = if(( cut_7 == 1 ) or ( cut_7 == 2 ); 3.3 mm; if(( cut_7 == 3 ) or ( cut_7 == 4 ) or ( cut_7 == 5 ); 2.7 mm; 2.125 mm))"
equation "parallel_distance_7 = if(( cut_7 == 1 ) or ( cut_7 == 2 ) or ( cut_7 == 3 ) or ( cut_7 == 4 ) or ( cut_7 == 5 ); 4.25 mm; 3.96625 mm)"
equation "pos_8 = round($8)"
equation "cut_8 = if(pos_8 == 1; 1; if(pos_8 == 2; 2; if(pos_8 == 3; 3; if(pos_8 == 4; 4; if(pos_8 == 5; 5; 6)))))"
equation "right_angle_8 = if(cut_8 == 1; 50 deg; if(cut_8 == 2; 65 deg; if(cut_8 == 3; 35 deg; if(cut_8 == 4; 50 deg; if(cut_8 == 5; 65 deg; 65 deg)))))"
equation "left_angle_8 = if(cut_8 == 1; 65 deg; if(cut_8 == 2; 50 deg; if(cut_8 == 3; 65 deg; if(cut_8 == 4; 50 deg; if(cut_8 == 5; 35 deg; 65 deg)))))"
equation "end_diameters_8 = if(( cut_8 == 1 ) or ( cut_8 == 2 ); 3.3 mm; if(( cut_8 == 3 ) or ( cut_8 == 4 ) or ( cut_8 == 5 ); 2.7 mm; 2.125 mm))"
equation "parallel_distance_8 = if(( cut_8 == 1 ) or ( cut_8 == 2 ) or ( cut_8 == 3 ) or ( cut_8 == 4 ) or ( cut_8 == 5 ); 4.25 mm; 3.96625 mm)"
equation "pos_9 = round($9)"
equation "cut_9 = if(pos_9 == 1; 1; if(pos_9 == 2; 2; if(pos_9 == 3; 3; if(pos_9 == 4; 4; if(pos_9 == 5; 5; 6)))))"
equation "right_angle_9 = if(cut_9 == 1; 50 deg; if(cut_9 == 2; 65 deg; if(cut_9 == 3; 35 deg; if(cut_9 == 4; 50 deg; if(cut_9 == 5; 65 deg; 65 deg)))))"
equation "left_angle_9 = if(cut_9 == 1; 65 deg; if(cut_9 == 2; 50 deg; if(cut_9 == 3; 65 deg; if(cut_9 == 4; 50 deg; if(cut_9 == 5; 35 deg; 65 deg)))))"
equation "end_diameters_9 = if(( cut_9 == 1 ) or ( cut_9 == 2 ); 3.3 mm; if(( cut_9 == 3 ) or ( cut_9 == 4 ) or ( cut_9 == 5 ); 2.7 mm; 2.125 mm))"
equation "parallel_distance_9 = if(( cut_9 == 1 ) or ( cut_9 == 2 ) or ( cut_9 == 3 ) or ( cut_9 == 4 ) or ( cut_9 == 5 ); 4.25 mm; 3.96625 mm)"
equation "d65 = d64"
equation "d67 = d66"
equation "d69 = d68"
equation "d70 = d68"
equation "d71 = d68"
equation "d73 = d72"
equation "d74 = d72"
equation "d75 = d72"
equation "d77 = d76"
equation "d79 = d78"
equation "d92 = d64"
equation "d93 = d64"
equation "d102 = ( 0.5 * 2.75 ) * 1 mm"
equation "d105 = ( 0.5 * 2.75 ) * 1 mm"
equation "d106 = 0.575 mm"
equation "d107 = 0.9 mm"
equation "d108 = 35 deg"
equation "d109 = -d106"
equation "d110 = -d107"
equation "d111 = d108"
equation "d112 = d76"
equation "d113 = d76"
equation "d116 = d115"
equation "d117 = d64 * 2.5"
equation "d118 = right_angle_1"
equation "d119 = left_angle_1"
equation "d120 = end_diameters_1"
equation "d121 = parallel_distance_1"
equation "d122 = parallel_distance_1"
equation "d123 = d117"
equation "d124 = right_angle_2"
equation "d125 = left_angle_2"
equation "d126 = end_diameters_2"
equation "d127 = parallel_distance_2"
equation "d128 = parallel_distance_2"
equation "d129 = d117"
equation "d130 = right_angle_3"
equation "d131 = left_angle_3"
equation "d132 = end_diameters_3"
equation "d133 = parallel_distance_3"
equation "d134 = parallel_distance_3"
equation "d135 = d117"
equation "d136 = right_angle_4"
equation "d137 = left_angle_4"
equation "d138 = end_diameters_4"
equation "d139 = parallel_distance_4"
equation "d140 = parallel_distance_4"
equation "d141 = d117"
equation "d142 = right_angle_5"
equation "d143 = left_angle_5"
equation "d144 = end_diameters_5"
equation "d145 = parallel_distance_5"
equation "d146 = parallel_distance_5"
equation "d147 = d117"
equation "d148 = right_angle_6"
equation "d149 = left_angle_6"
equation "d150 = end_diameters_6"
equation "d151 = parallel_distance_6"
equation "d152 = parallel_distance_6"
equation "d153 = d117"
equation "d154 = right_angle_7"
equation "d155 = left_angle_7"
equation "d156 = end_diameters_7"
equation "d157 = parallel_distance_7"
equation "d158 = parallel_distance_7"
equation "d159 = d117"
equation "d160 = right_angle_8"
equation "d161 = left_angle_8"
equation "d162 = end_diameters_8"
equation "d163 = parallel_distance_8"
equation "d164 = parallel_distance_8"
equation "d165 = d117"
equation "d166 = right_angle_9"
equation "d167 = left_angle_9"
equation "d168 = end_diameters_9"
equation "d169 = parallel_distance_9"
equation "d170 = parallel_distance_9"
equation "d171 = d117"
equation "d174 = -2.07 mm - ( 1.5 * 1 mm )"
equation "d177 = -2.07 mm - ( 1.5 * 2 mm )"
equation "d180 = -2.07 mm - ( 1.5 * 3 mm )"
equation "d183 = -2.07 mm - ( 1.5 * 4 mm )"
equation "d186 = -2.07 mm - ( 1.5 * 5 mm )"
equation "d189 = -2.07 mm - ( 1.5 * 6 mm )"
equation "d192 = -2.07 mm - ( 1.5 * 8 mm )"
equation "d195 = -2.07 mm - ( 1.5 * 9 mm )"
equation "d198 = -2.07 mm - ( 1.5 * 10 mm )"
equation "d201 = d106"
equation "d202 = d107"
equation "d203 = d108"
equation "d204 = -d106"
equation "d205 = -d107"
equation "d206 = d108"
